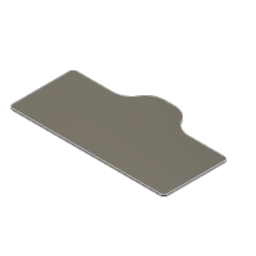
Culture Retainer Wall v2 (Autodesk Fusion 360 design; units mm, degrees)
Autodesk Fusion 360 part; units mm, degrees
sketch "Sketch1" plane through (0, 0, 0) normal (0, 1, 0) x (1, 0, 0)
  line L0 (0, 0) -> (82, 0)
  line L1 (82, 0) -> (82, 34)
  line L2 (82, 34) -> (0, 34)
  line L3 (0, 34) -> (0, 0)
  line L4 (31, 44) -> (51, 44)
  line L5 (51, 44) -> (51, 34)
  line L6 (51, 34) -> (31, 34)
  line L7 (31, 34) -> (31, 44)
  dimension "d1" = 82
  dimension "d2" = 34
  dimension "d3" = 20
  dimension "d4" = 10
  constraint horizontal L0
  constraint vertical L1
  constraint horizontal L2
  constraint vertical L3
  constraint coincident L0.start L3.end
  constraint horizontal L4
  constraint vertical L5
  constraint horizontal L6
  constraint vertical L7
  constraint midpoint L2 L6
  measures "d1" distance of L1.end L2.end
  measures "d2" distance of L0.start L2.end
  measures "d3" distance of L4.start L4.end
  measures "d4" distance of L4.end L5.end
extrude "Extrude1" add sketch "Sketch1" along normal blind 1
fillet "Fillet1" radius 10 4 edges at (51, 0.5, -34) (51, 0.5, -44) (31, 0.5, -44) (31, 0.5, -34)
fillet "Fillet2" radius 2 4 edges at (0, 0.5, 0) (82, 0.5, 0) (82, 0.5, -34) (0, 0.5, -34)
